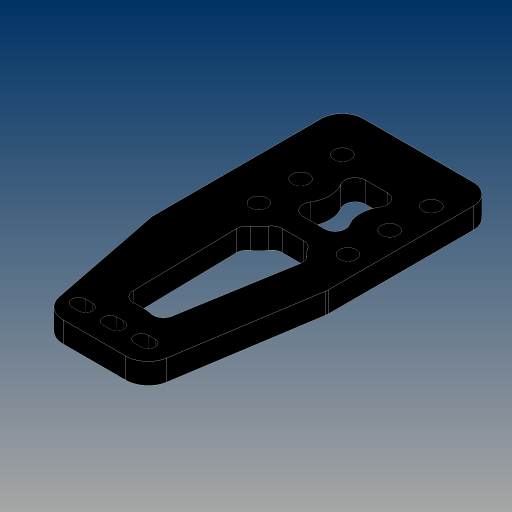
# Autodesk Inventor part: ELEV_025_CHAINCLAMP1
Saved by Autodesk Inventor 2024.3 (Build 283343000, 343)
## iProperties
Created: 2024-11-28
Part Number: ELEV_025_CHAINCLAMP1
Material: Aluminum 6061
Document SubType Name: Modeling
Designer: Kenji
Density: 2.7 g/cm^3
Appearance: Anodized - Black
Mass: 53.6652 g
Surface Area: 99.507 cm^2
Volume: 19.876 cm^3
Author: Kenji
Autodesk Inventor part; units mm, degrees
ref_plane "YZ Plane" through (0, 0, 0) normal (1, 0, 0) x (0, 1, 0)
ref_plane "XZ Plane" through (0, 0, 0) normal (0, 1, 0) x (-1, 0, 0)
ref_plane "XY Plane" through (0, 0, 0) normal (0, 0, 1) x (1, 0, 0)
sketch "Sketch1" plane through (0, 0, 0) normal (0, 1, 0) x (-1, 0, 0)
  line L0 (0, 25.4) -> (0, -25.4) construction
  line L1 (0, -25.4) -> (46.1518, -25.4) construction
  line L2 (15.4178, 64.3509) -> (13.335, 64.3509)
  line L3 (15.4178, 68.5165) -> (13.335, 68.5165)
  arc A0 (13.335, 68.5165) -> (13.335, 64.3509) centre (13.335, 66.4337) ccw
  arc A1 (15.4178, 64.3509) -> (15.4178, 68.5165) centre (15.4178, 66.4337) ccw
  circle A2 centre (13.335, 66.4337) radius 6.8266 construction
  line L4 (32.385, 73.2603) -> (13.335, 73.2603)
  circle A3 centre (6.35, 0) radius 2.54
  circle A4 centre (6.35, -12.7) radius 2.54
  circle A5 centre (6.35, 12.7) radius 2.54
  line L5 (6.35, -12.7) -> (6.35, 12.7) construction
  line L6 (6.5905, 67.4898) -> (0.0764, 25.8882)
  line L7 (0, 24.9059) -> (0, -19.05)
  arc A6 (0.0764, 25.8882) -> (0, 24.9059) centre (6.35, 24.9059) ccw
  line L8 (46.1518, -19.05) -> (46.1518, 31.75)
  line L9 (39.0793, 67.7714) -> (46.0287, 32.9943)
  arc A7 (46.1518, 31.75) -> (46.0287, 32.9943) centre (39.8018, 31.75) ccw
  arc A8 (13.335, 73.2603) -> (6.5905, 67.4898) centre (13.335, 66.4337) ccw
  line L10 (39.8018, -25.4) -> (6.35, -25.4)
  circle A9 centre (33.4518, 12.7) radius 2.54
  circle A10 centre (33.4518, 0) radius 2.54
  circle A11 centre (33.4518, -12.7) radius 2.54
  line L11 (33.4518, -12.7) -> (33.4518, 12.7) construction
  arc A12 (39.8018, -25.4) -> (46.1518, -19.05) centre (39.8018, -19.05) ccw
  arc A13 (0, -19.05) -> (6.35, -25.4) centre (6.35, -19.05) ccw
  arc A14 (24.9428, 64.3509) -> (24.9428, 68.5165) centre (24.9428, 66.4337) ccw
  line L12 (24.9428, 64.3509) -> (22.86, 64.3509)
  line L13 (24.9428, 68.5165) -> (22.86, 68.5165)
  arc A15 (22.86, 68.5165) -> (22.86, 64.3509) centre (22.86, 66.4337) ccw
  circle A16 centre (22.86, 66.4337) radius 6.8266 construction
  arc A17 (34.4678, 64.3509) -> (34.4678, 68.5165) centre (34.4678, 66.4337) ccw
  line L14 (34.4678, 64.3509) -> (32.385, 64.3509)
  line L15 (34.4678, 68.5165) -> (32.385, 68.5165)
  arc A18 (32.385, 68.5165) -> (32.385, 64.3509) centre (32.385, 66.4337) ccw
  circle A19 centre (32.385, 66.4337) radius 6.8266 construction
  arc A20 (39.0793, 67.7714) -> (32.385, 73.2603) centre (32.385, 66.4337) ccw
  line L16 (34.4678, 66.4337) -> (13.335, 66.4337) construction
  point P0 (0, 0)
  point P1 (0, 0)
  point P2 (22.86, 73.2603)
  point P3 (16.1155, 67.4898)
  point P4 (25.6405, 67.4898)
  dimension "d2" = 50.8
  dimension "d3" = 6.35
  dimension "d6" = 91.8337
  dimension "d8" = 13.335
  dimension "d9" = 2.0828
  dimension "d10" = 2.0828
  dimension "d11" = 2.0828
  dimension "d21" = 13.6533
  dimension "d31" = 5.08
  dimension "d32" = 12.7
  dimension "d33" = 12.7
  dimension "d41" = 6.35
  dimension "d42" = 6.35
  dimension "d43" = 13.335
  dimension "d45" = 12.7
  dimension "d46" = 12.7
  dimension "d47" = 6.35
  dimension "d85" = 9.525
  dimension "d90" = 27.1018
  constraints: 34 end point, 32 point on circle, 21 centre point, 14 tangent, 8 equal radius, 6 point on line, 4 coincident, 4 horizontal alignment, 4 midpoint, 4 parallel, 4 vertical, 3 horizontal, 2 collinear, 28 other
  measures "d2" distance of L0.start L0.end
  measures "d3" distance from line of L0 point (6.35, 0)
  measures "d6" distance from line of L1 A0.centre
  measures "d8" distance from line of L0 A0.centre
  measures "d9" radius of A1
  measures "d10" radius of A0
  measures "d11" distance of L2.start L2.end
  measures "d21" diameter of A2
  measures "d31" diameter of A3
  measures "d32" distance of L5.end A3.centre
  measures "d33" distance of L5.start A3.centre
  measures "d41" radius of A6
  measures "d42" radius of A7
  measures "d43" distance from line of L0 A2.centre
  measures "d45" distance of L11.start A10.centre
  measures "d46" distance from line of L8 L11.end
  measures "d47" radius of A12
  measures "d85" distance of A1.centre A14.centre
  measures "d90" distance of L5.end L11.end
extrude "Extrusion3" add sketch "Sketch1" along normal blind 6.35
sketch "Sketch3" plane through (0, 6.35, 0) normal (0, 1, 0) x (1, 0, 0)
  line L0 (-32.385, -73.2603) -> (-13.335, -73.2603) construction
  arc A0 (-13.335, -73.2603) -> (-6.5905, -67.4898) centre (-13.335, -66.4337) ccw construction
  line L1 (-6.5905, -67.4898) -> (-0.0764, -25.8882) construction
  arc A1 (-0.0764, -25.8882) -> (0, -24.9059) centre (-6.35, -24.9059) ccw construction
  line L2 (0, -24.9059) -> (0, 19.05) construction
  arc A2 (0, 19.05) -> (-6.35, 25.4) centre (-6.35, 19.05) ccw construction
  line L3 (-6.35, 25.4) -> (-39.8018, 25.4) construction
  arc A3 (-39.8018, 25.4) -> (-46.1518, 19.05) centre (-39.8018, 19.05) ccw construction
  line L4 (-46.1518, 19.05) -> (-46.1518, -31.75) construction
  arc A4 (-46.1518, -31.75) -> (-46.0287, -32.9943) centre (-39.8018, -31.75) ccw construction
  line L5 (-46.0287, -32.9943) -> (-39.0793, -67.7714) construction
  arc A5 (-39.0793, -67.7714) -> (-32.385, -73.2603) centre (-32.385, -66.4337) ccw construction
  circle A6 centre (-6.35, 0) radius 2.54 construction
  circle A7 centre (-6.35, 12.7) radius 2.54 construction
  circle A8 centre (-6.35, -12.7) radius 2.54 construction
  circle A9 centre (-33.4518, -12.7) radius 2.54 construction
  circle A10 centre (-33.4518, 0) radius 2.54 construction
  circle A11 centre (-33.4518, 12.7) radius 2.54 construction
  line L6 (-34.4678, -64.3509) -> (-32.385, -64.3509) construction
  arc A12 (-32.385, -68.5165) -> (-32.385, -64.3509) centre (-32.385, -66.4337) ccw construction
  line L7 (-32.385, -68.5165) -> (-34.4678, -68.5165) construction
  arc A13 (-34.4678, -64.3509) -> (-34.4678, -68.5165) centre (-34.4678, -66.4337) ccw construction
  line L8 (-24.9428, -64.3509) -> (-22.86, -64.3509) construction
  arc A14 (-22.86, -68.5165) -> (-22.86, -64.3509) centre (-22.86, -66.4337) ccw construction
  line L9 (-22.86, -68.5165) -> (-24.9428, -68.5165) construction
  arc A15 (-24.9428, -64.3509) -> (-24.9428, -68.5165) centre (-24.9428, -66.4337) ccw construction
  arc A16 (-15.4178, -64.3509) -> (-15.4178, -68.5165) centre (-15.4178, -66.4337) ccw construction
  line L10 (-15.4178, -64.3509) -> (-13.335, -64.3509) construction
  arc A17 (-13.335, -68.5165) -> (-13.335, -64.3509) centre (-13.335, -66.4337) ccw construction
  line L11 (-13.335, -68.5165) -> (-15.4178, -68.5165) construction
  line L12 (-32.8524, -66.5271) -> (-39.8018, -31.75) construction
  line L13 (-39.8018, -31.75) -> (-39.8018, 19.05) construction
  line L14 (-39.8018, 19.05) -> (-6.35, 19.05) construction
  line L15 (-6.35, 19.05) -> (-6.35, -24.9059) construction
  line L16 (-6.35, -24.9059) -> (-12.8641, -66.5074) construction
  arc A18 (-13.335, -66.9103) -> (-12.8641, -66.5074) centre (-13.335, -66.4337) ccw construction
  line L17 (-13.335, -66.9103) -> (-32.385, -66.9103) construction
  arc A19 (-32.8524, -66.5271) -> (-32.385, -66.9103) centre (-32.385, -66.4337) ccw construction
  line L18 (-34.4678, -74.8665) -> (-32.385, -74.8665) construction
  arc A20 (-32.385, -74.8665) -> (-32.385, -58.0009) centre (-32.385, -66.4337) ccw construction
  line L19 (-32.385, -58.0009) -> (-34.4678, -58.0009) construction
  arc A21 (-34.4678, -58.0009) -> (-34.4678, -74.8665) centre (-34.4678, -66.4337) ccw construction
  line L20 (-24.9428, -74.8665) -> (-22.86, -74.8665) construction
  arc A22 (-22.86, -74.8665) -> (-22.86, -58.0009) centre (-22.86, -66.4337) ccw construction
  line L21 (-22.86, -58.0009) -> (-24.9428, -58.0009) construction
  arc A23 (-24.9428, -58.0009) -> (-24.9428, -74.8665) centre (-24.9428, -66.4337) ccw construction
  arc A24 (-15.4178, -58.0009) -> (-15.4178, -74.8665) centre (-15.4178, -66.4337) ccw construction
  line L22 (-15.4178, -58.0009) -> (-13.335, -58.0009) construction
  arc A25 (-13.335, -74.8665) -> (-13.335, -58.0009) centre (-13.335, -66.4337) ccw construction
  line L23 (-13.335, -74.8665) -> (-15.4178, -74.8665) construction
  circle A26 centre (-33.4518, -12.7) radius 8.89 construction
  circle A27 centre (-33.4518, 0) radius 8.89 construction
  circle A28 centre (-33.4518, 12.7) radius 8.89 construction
  circle A29 centre (-6.35, 12.7) radius 8.89 construction
  circle A30 centre (-6.35, 0) radius 8.89 construction
  circle A31 centre (-6.35, -12.7) radius 8.89 construction
  line L24 (-24.5618, -12.7) -> (-15.24, -12.7) construction
  line L25 (-24.5618, 12.7) -> (-15.24, 12.7) construction
  line L26 (-32.5524, -58.0009) -> (-33.2753, -21.5882) construction
  line L27 (-13.9947, -58.0009) -> (-7.8293, -21.4661) construction
  line L28 (-29.4371, -54.9642) -> (-30.0738, -22.8937)
  line L29 (-16.8301, -55.7221) -> (-11.1878, -22.2874)
  line L30 (-23.1931, -15.875) -> (-16.6087, -15.875)
  line L31 (-23.1931, -9.525) -> (-16.6087, -9.525)
  line L32 (-23.1931, 9.525) -> (-16.6087, 9.525)
  arc A32 (-28.6237, -20.1647) -> (-25.8927, -17.3789) centre (-33.4518, -12.7) ccw
  arc A33 (-13.9091, -17.3789) -> (-12.2216, -19.3751) centre (-6.35, -12.7) ccw
  arc A34 (-28.6237, -20.1647) -> (-30.0738, -22.8937) centre (-26.8994, -22.8307) ccw
  arc A35 (-23.1931, -15.875) -> (-25.8927, -17.3789) centre (-23.1931, -19.05) ccw
  arc A36 (-13.9091, -17.3789) -> (-16.6087, -15.875) centre (-16.6087, -19.05) ccw
  arc A37 (-11.1878, -22.2874) -> (-12.2216, -19.3751) centre (-14.3185, -21.7591) ccw
  arc A38 (-25.8927, -4.6789) -> (-25.8927, 4.6789) centre (-33.4518, 0) ccw
  arc A39 (-13.9091, 4.6789) -> (-13.9091, -4.6789) centre (-6.35, 0) ccw
  arc A40 (-13.9091, -8.0211) -> (-13.9091, -8.0211) centre (-6.35, -12.7) ccw
  arc A41 (-25.8927, -8.0211) -> (-25.8927, -8.0211) centre (-33.4518, -12.7) ccw
  arc A42 (-25.8927, 8.0211) -> (-25.8927, 8.0211) centre (-33.4518, 12.7) ccw
  arc A43 (-13.9091, 8.0211) -> (-13.9091, 8.0211) centre (-6.35, 12.7) ccw
  arc A44 (-25.8927, -8.0211) -> (-23.1931, -9.525) centre (-23.1931, -6.35) ccw
  arc A45 (-25.8927, -4.6789) -> (-25.8927, -8.0211) centre (-23.1931, -6.35) ccw
  arc A46 (-23.1931, 9.525) -> (-25.8927, 8.0211) centre (-23.1931, 6.35) ccw
  arc A47 (-25.8927, 8.0211) -> (-25.8927, 4.6789) centre (-23.1931, 6.35) ccw
  arc A48 (-13.9091, 8.0211) -> (-16.6087, 9.525) centre (-16.6087, 6.35) ccw
  arc A49 (-13.9091, 4.6789) -> (-13.9091, 8.0211) centre (-16.6087, 6.35) ccw
  arc A50 (-16.6087, -9.525) -> (-13.9091, -8.0211) centre (-16.6087, -6.35) ccw
  arc A51 (-13.9091, -8.0211) -> (-13.9091, -4.6789) centre (-16.6087, -6.35) ccw
  arc A52 (-24.9428, -58.0009) -> (-25.9017, -58.0556) centre (-24.9428, -66.4337) ccw
  arc A53 (-20.7538, -58.2682) -> (-22.86, -58.0009) centre (-22.86, -66.4337) ccw
  arc A54 (-17.2486, -58.202) -> (-19.1389, -58.8663) centre (-15.4178, -66.4337) ccw
  arc A55 (-28.6639, -58.8663) -> (-29.3657, -58.56) centre (-32.385, -66.4337) ccw
  arc A56 (-29.4371, -54.9642) -> (-25.9017, -58.0556) centre (-26.2627, -54.9012) ccw
  arc A57 (-20.7538, -58.2682) -> (-16.8301, -55.7221) centre (-19.9608, -55.1938) ccw
  line L33 (-24.9428, -58.0009) -> (-22.86, -58.0009)
  point P0 (0, 0)
  point P1 (-30.1126, -20.939)
  point P2 (-10.8625, -20.3596)
  point P3 (-25.1481, -15.875)
  point P4 (-14.6537, -15.875)
  point P5 (-25.1481, -9.525)
  point P6 (-14.6537, -9.525)
  point P7 (-25.1481, 9.525)
  point P8 (-14.6537, 9.525)
  point P9 (-13.9091, 8.0211)
  point P10 (-25.8927, 8.0211)
  dimension "d93" = 6.35
  dimension "d94" = 6.35
  dimension "d95" = 6.35
  dimension "d96" = 6.35
  dimension "d97" = 6.35
  dimension "d98" = 6.35
  dimension "d99" = 6.35
  dimension "d100" = 6.35
  dimension "d101" = 6.35
  dimension "d102" = 6.35
  dimension "d104" = 3.175
  dimension "d105" = 3.175
  dimension "d107" = 3.175
  dimension "d108" = 3.175
  dimension "d109" = 3.175
  dimension "d112" = 3.175
  dimension "d113" = 3.175
  dimension "d114" = 3.175
  dimension "d115" = 3.175
  dimension "d116" = 3.175
  dimension "d119" = 3.175
  constraints: 98 point on circle, 44 end point, 40 centre point, 33 tangent, 20 equal radius, 18 point on line, 6 parallel, 2 concentric, 1 horizontal, 16 other
  measures "d93" distance between parallel lines of L5 L12
  measures "d94" radial gap between concentric circles of A13 A21
  measures "d95" radial gap between concentric circles of A15 A23
  measures "d96" radial gap between concentric circles of A16 A24
  measures "d97" radial gap between concentric circles of A9 A26
  measures "d98" radial gap between concentric circles of A10 A27
  measures "d99" radial gap between concentric circles of A11 A28
  measures "d100" radial gap between concentric circles of A7 A29
  measures "d101" radial gap between concentric circles of A6 A30
  measures "d102" radial gap between concentric circles of A8 A31
  measures "d104" distance between parallel lines of L26 L28
  measures "d105" distance between parallel lines of L27 L29
  measures "d107" distance between parallel lines of L24 L30
  measures "d108" distance between parallel lines of L24 L31
  measures "d109" distance between parallel lines of L25 L32
  measures "d112" radius of A34
  measures "d113" radius of A37
  measures "d114" radius of A44
  measures "d115" radius of A46
  measures "d116" radius of A48
  measures "d119" radius of A56
extrude "Extrusion5" cut sketch "Sketch3" against normal blind 25.4 contours L28 A34 A32 A35 L30 A36 A33 A37 L29 A57 A53 L33 A52 A56 | A45 A38 A47 A46 L32 A48 A49 A39 A51 A50 L31 A44
body "Solid2"
